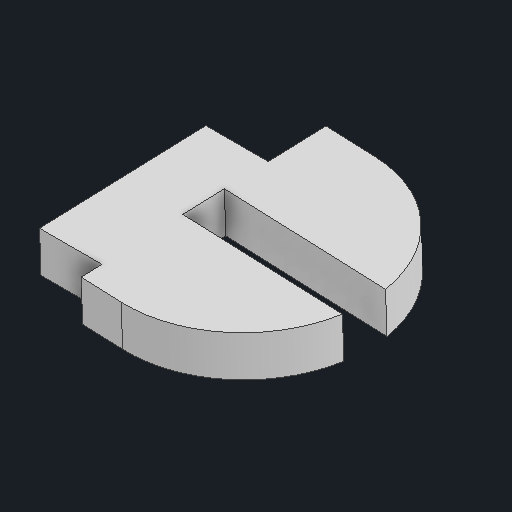
# Autodesk Inventor part: sponson_spanner_side_holder
Saved by Autodesk Inventor 2023 (Build 270158030, 158C)
## iProperties
Created: 2022-03-22
Part Number: sponson_spanner_side_holder
Material: Generic
Document SubType Name: Modeling
Designer: kardo
Density: 1 g/cm^3
Appearance: Default
Author: kardo
Autodesk Inventor part; units mm, degrees
ref_plane "YZ Plane" through (0, 0, 0) normal (1, 0, 0) x (0, 1, 0)
ref_plane "XZ Plane" through (0, 0, 0) normal (0, 1, 0) x (-1, 0, 0)
ref_plane "XY Plane" through (0, 0, 0) normal (0, 0, 1) x (1, 0, 0)
derived "parameters_frame.ipt"
derived "surface_body.ipt"
ref_plane "plane_tunnel_right" through (81.12, 0, 0) normal (1, 0, 0) x (0, 1, 0)
ref_plane "plane_sponson_side" through (81.12, 237, 36.448) normal (0.0378267, 0.0348745, -0.9986756) x (0.3011979, -0.9533106, -0.0218819)
derived "stencil_frame.ipt"
sketch "sk_joint_locations" plane through (81.12, 0, 0) normal (1, 0, 0) x (0, 1, 0)
  line L0 (0, 0) -> (111.39, 7.7891) construction
  line L1 (30.81, 28.832) -> (94.8, 28.832) construction
  arc A0 (30.81, 28.832) -> (9.48, 28.5282) centre (30.81, -720.1791) ccw construction
  line L2 (-254.1001, 21.0191) -> (9.48, 28.5282) construction
  line L3 (-363, 18.496) -> (-275.8801, 20.463) construction
  arc A1 (-275.8801, 20.463) -> (-254.1001, 21.0191) centre (-359.1231, 3707.4463) ccw construction
  line L4 (-215.9778, 4689.3669) -> (255.6105, -2054.6605) construction
  line L5 (-242.0001, 4666.1952) -> (-242.0001, -2045.0469) construction
  line L6 (-120.9999, 4666.1952) -> (-120.9999, -2045.0469) construction
  line L7 (-363, 4666.1952) -> (-363, -2045.0469) construction
  line L8 (0, 4666.1952) -> (0, -2045.0469) construction
  line L9 (554.3783, 47.5311) -> (-618.9921, 6.5561) construction
  line L10 (-688.3759, -28.2606) -> (714.4996, 69.838) construction
  line L11 (178.2183, 30.3929) -> (177.9391, 38.388) construction
  line L12 (185.9231, 36.8959) -> (186.4825, 28.8959) construction
  line L13 (0, 8.704) -> (111.0257, 12.9988) construction
  line L14 (-242.0001, 45.8501) -> (-242.0001, 21.3638) construction
  line L15 (-363, 37.4293) -> (-363, 18.496) construction
  line L16 (-120.9999, 51.0063) -> (-120.9999, 24.811) construction
  line L17 (0, 52.89) -> (0, 28.2581) construction
  line L18 (108.3896, 50.6971) -> (108.9168, 43.1574) construction
  line L19 (109.444, 35.6178) -> (108.9168, 43.1574) construction
  line L20 (109.444, 35.6178) -> (109.9713, 28.0781) construction
  line L21 (109.9713, 28.0781) -> (110.4985, 20.5385) construction
  line L22 (110.4985, 20.5385) -> (111.0257, 12.9988) construction
  line L23 (0, 8.704) -> (0, 0) construction
  line L24 (94.8, 37.536) -> (94.8, 28.832) construction
  line L25 (94.8, 35.548) -> (94.8, 30.82) construction
  spline S0 degree 4 poles (-363, 37.4293) (-272.3626, 45.1427) (-181.5879, 49.7528) (-90.8131, 52.89) (0, 52.89) knots 0 0 0 0 0 1 1 1 1 1
  spline S1 degree 3 poles (0, 52.89) (86.3106, 52.89) (181.3207, 49.5034) (237, 36.448) knots 0 0 0 0 1 1 1 1
  spline S2 degree 2 poles (111.39, 7.7891) (176.0348, 12.3096) (237, 36.448) knots 0 0 0 1 1 1
  point P0 (-215.9778, 4689.3669)
  point P1 (255.6105, -2054.6605)
  point P2 (178.0787, 34.3904)
  point P3 (186.2028, 32.8959)
  point P4 (134.9575, 11.3411)
  point P5 (-363, 27.9627)
  point P6 (-242.0001, 33.6069)
  point P7 (-120.9999, 37.9086)
  point P8 (0, 40.5741)
  point P9 (94.8, 33.184)
ref_plane "plane_base" through (81.12, 178.0787, 34.3904) normal (0, -0.9993908, -0.0348995) x (1, 0, 0)
sketch "sk_base" plane through (81.12, 178.0787, 34.3904) normal (0, -0.9993908, -0.0348995) x (1, 0, 0)
  line L0 (0, 4579.0534) -> (0, -1645.4832) projected
  line L1 (202.8549, 7.6788) -> (-161.6647, -6.1196) construction
  line L2 (11.0521, -1.5831) -> (3, -1.8879)
  line L3 (3, -1.8879) -> (3, 0.1136)
  line L4 (3, 0.1136) -> (10.9765, 0.4155)
  line L5 (0, 4) -> (3, 4)
  line L6 (3, 4) -> (3, 5)
  line L7 (3, 5) -> (4.9986, 5.0757)
  line L8 (0, -4) -> (3, -4)
  line L9 (3, -4) -> (3, -6.7743)
  line L10 (3, -6.7743) -> (5.4436, -6.6818)
  arc A0 (5.4436, -6.6818) -> (4.9986, 5.0757) centre (5.2211, -0.8031) ccw
  line L11 (3, -0.8872) -> (11.0998, -0.5805) construction
  line L12 (4.9986, 5.0757) -> (5.4436, -6.6818) construction
  point P0 (-81.12, -28.1546)
  dimension "d3" = 3
  dimension "d4" = 2
  dimension "d5" = 2
  dimension "d6" = 1
  constraints: 22 end point, 5 parallel, 5 point on circle, 3 collinear, 2 perpendicular, 2 tangent, 1 centre point, 1 midpoint, 1 point on line
  measures "d3" distance between parallel lines of L0 L6
  measures "d4" distance between parallel lines of L1 L2
  measures "d5" distance of L6.end L7.end
  measures "d6" distance of L5.end L6.end
extrude "thicken" add sketch "sk_base" along normal blind 2 contours L5 L6 L7 A0 L4 L3 L2 L10 L9 L8 L0
equation "\"d3\" = stringer_thickness"
equation "\"d4\" = bulkhead_thickness"
equation "\"d5\" = bulkhead_thickness"
equation "\"d6\" = 0.5 * bulkhead_thickness"
equation "\"d7\" = bulkhead_thickness"
equation "\"stringer_thickness\" = 3"
equation "\"bulkhead_thickness\" = 2"
body "Solid1"
